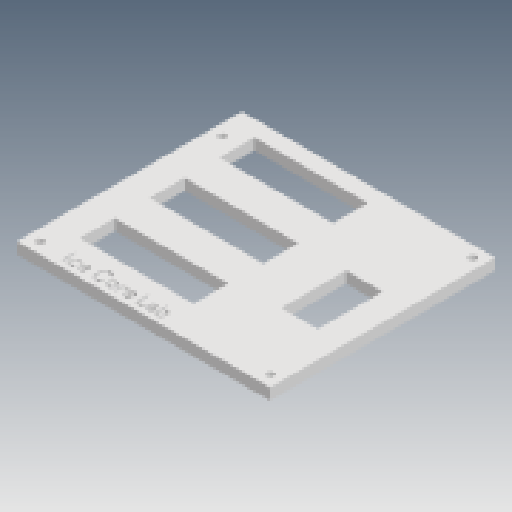
# Autodesk Inventor part: base_plate
Saved by Autodesk Inventor 2025.1 (Build 291241000, 241)
## iProperties
Created: 2026-06-20
Part Number: base_plate
Material: Generic
Document SubType Name: Modeling
Designer: Aiden
Density: 1 g/cm^3
Appearance: Default
Author: Aiden
Autodesk Inventor part; units mm, degrees
ref_plane "YZ Plane" through (0, 0, 0) normal (1, 0, 0) x (0, 1, 0)
ref_plane "XZ Plane" through (0, 0, 0) normal (0, 1, 0) x (-1, 0, 0)
ref_plane "XY Plane" through (0, 0, 0) normal (0, 0, 1) x (1, 0, 0)
sketch "Sketch1" plane through (0, 0, 0) normal (0, 1, 0) x (-1, 0, 0)
  line L0 (112.5, 100) -> (-112.5, 100)
  line L1 (-112.5, 100) -> (-112.5, -100)
  line L2 (-112.5, -100) -> (112.5, -100)
  line L3 (112.5, -100) -> (112.5, 100)
  line L4 (112.5, 100) -> (-112.5, -100) construction
  line L5 (-112.5, 100) -> (112.5, -100) construction
  point P0 (0, 0)
  dimension "d0" = 200
  dimension "d1" = 225
  constraints: 12 end point, 2 midpoint, 2 parallel, 1 horizontal, 1 perpendicular
  measures "d0" distance of L2.end L0.start
  measures "d1" distance of L1.end L2.end
extrude "Extrusion1" add sketch "Sketch1" along normal blind 10
sketch "Sketch3" plane through (0, 10, 0) normal (0, 1, 0) x (1, 0, 0)
  line L0 (-86.9553, 54.5452) -> (13.9553, 54.5452)
  line L1 (13.9553, 54.5452) -> (13.9553, 85.4548)
  line L2 (13.9553, 85.4548) -> (-86.9553, 85.4548)
  line L3 (-86.9553, 85.4548) -> (-86.9553, 54.5452)
  line L4 (-86.9553, 54.5452) -> (13.9553, 85.4548) construction
  line L5 (13.9553, 54.5452) -> (-86.9553, 85.4548) construction
  line L6 (-112.5, 100) -> (-112.5, -100) projected
  line L7 (112.5, 100) -> (-112.5, 100) projected
  line L8 (-86.9553, 23.4548) -> (-86.9553, -7.4548)
  line L9 (-86.9553, -7.4548) -> (13.9553, -7.4548)
  line L10 (13.9553, 23.4548) -> (-86.9553, 23.4548)
  line L11 (13.9553, -7.4548) -> (13.9553, 23.4548)
  line L12 (-86.9553, -38.5452) -> (-86.9553, -69.4548)
  line L13 (-86.9553, -69.4548) -> (13.9553, -69.4548)
  line L14 (13.9553, -38.5452) -> (-86.9553, -38.5452)
  line L15 (13.9553, -69.4548) -> (13.9553, -38.5452)
  point P0 (0, 0)
  point P1 (-36.5, 70)
  dimension "d6" = 76
  dimension "d7" = 30
  dimension "d10" = 62
  constraints: 28 end point, 2 midpoint, 2 parallel, 1 collinear, 1 horizontal, 1 perpendicular, 1 vertical, 15 other
  measures "d6" distance from line of L6 point (-36.5, 70)
  measures "d7" distance from line of L7 point (-36.5, 70)
  measures "d10" distance of L2.end L8.start
extrude "Extrusion3" cut sketch "Sketch3" against normal through all
sketch "Sketch4" plane through (0, 10, 0) normal (0, 1, 0) x (1, 0, 0)
  line L0 (56.2706, -33.7574) -> (88.7294, -33.7574)
  line L1 (88.7294, -33.7574) -> (88.7294, 23.7574)
  line L2 (88.7294, 23.7574) -> (56.2706, 23.7574)
  line L3 (56.2706, 23.7574) -> (56.2706, -33.7574)
  line L4 (56.2706, -33.7574) -> (88.7294, 23.7574) construction
  line L5 (88.7294, -33.7574) -> (56.2706, 23.7574) construction
  line L6 (112.5, -100) -> (112.5, 100) projected
  line L7 (-112.5, -100) -> (112.5, -100) projected
  point P0 (0, 0)
  point P1 (72.5, -5)
  dimension "d17" = 40
  dimension "d18" = 95
  constraints: 12 end point, 2 midpoint, 2 parallel, 1 horizontal, 1 perpendicular
  measures "d17" distance from line of L6 point (72.5, -5)
  measures "d18" distance from line of L7 point (72.5, -5)
extrude "Extrusion4" cut sketch "Sketch4" against normal through all
sketch "Sketch2" plane through (0, 10, 0) normal (0, 1, 0) x (1, 0, 0)
  line L0 (-13.404, -88.2397) -> (-13.404, -81.8012)
  line L1 (-13.404, -81.8012) -> (-13.1143, -82.3338)
  line L2 (-13.1143, -82.3338) -> (-12.6963, -83.0794)
  line L3 (-12.6963, -83.0794) -> (-12.6242, -83.2099)
  line L4 (-12.6242, -83.2099) -> (-12.581, -83.3384)
  line L5 (-12.581, -83.3384) -> (-12.5534, -83.5231)
  line L6 (-12.5534, -83.5231) -> (-12.5284, -83.822)
  line L7 (-12.5284, -83.822) -> (-12.451, -84.7515)
  line L8 (-12.451, -84.7515) -> (-12.3895, -85.418)
  line L9 (-12.3895, -85.418) -> (-12.3583, -85.6558)
  line L10 (-12.3583, -85.6558) -> (-12.3386, -85.6951)
  line L11 (-12.3386, -85.6951) -> (-12.313, -85.6763)
  line L12 (-12.313, -85.6763) -> (-12.2357, -85.4495)
  line L13 (-12.2357, -85.4495) -> (-12.1082, -84.945)
  line L14 (-12.1082, -84.945) -> (-11.9568, -84.3511)
  line L15 (-11.9568, -84.3511) -> (-11.879, -84.1041)
  line L16 (-11.879, -84.1041) -> (-11.6102, -84.3782)
  line L17 (-11.6102, -84.3782) -> (-11.3666, -84.6522)
  line L18 (-11.3666, -84.6522) -> (-11.3476, -88.7862)
  line L19 (-11.3476, -88.7862) -> (-11.3285, -92.9202)
  line L20 (-11.3285, -92.9202) -> (-9.2689, -92.93)
  line L21 (-9.2689, -92.93) -> (-7.2093, -92.9399)
  line L22 (-7.2093, -92.9399) -> (-6.7745, -93.3469)
  line L23 (-6.7745, -93.3469) -> (-5.8675, -94.2035)
  line L24 (-5.8675, -94.2035) -> (-5.3953, -94.6529)
  line L25 (-5.3953, -94.6529) -> (-9.314, -94.6561)
  line L26 (-9.314, -94.6561) -> (-13.3183, -94.6688)
  line L27 (-13.3183, -94.6688) -> (-13.3466, -94.6593)
  line L28 (-13.3466, -94.6593) -> (-13.3679, -94.5737)
  line L29 (-13.3679, -94.5737) -> (-13.3933, -93.8723)
  line L30 (-13.3933, -93.8723) -> (-13.404, -88.2397)
  line L31 (-3.7121, -94.6461) -> (-4.5026, -93.8769)
  line L32 (-4.5026, -93.8769) -> (-5.255, -93.1487)
  line L33 (-5.255, -93.1487) -> (-5.2617, -92.2745)
  line L34 (-5.2617, -92.2745) -> (-5.2684, -91.4003)
  line L35 (-5.2684, -91.4003) -> (-4.4522, -90.6105)
  line L36 (-4.4522, -90.6105) -> (-3.7551, -89.9567)
  line L37 (-3.7551, -89.9567) -> (-3.5944, -89.8366)
  line L38 (-3.5944, -89.8366) -> (-3.4895, -89.7956)
  line L39 (-3.4895, -89.7956) -> (-2.9007, -89.7861)
  line L40 (-2.9007, -89.7861) -> (-1.6907, -89.7986)
  line L41 (-1.6907, -89.7986) -> (-0.4099, -89.8104)
  line L42 (-0.4099, -89.8104) -> (-0.103, -89.8024)
  line L43 (-0.103, -89.8024) -> (0.0122, -89.7849)
  line L44 (0.0122, -89.7849) -> (0.0351, -89.7449)
  line L45 (0.0351, -89.7449) -> (0.0486, -89.6654)
  line L46 (0.0486, -89.6654) -> (0.0502, -89.3514)
  line L47 (0.0502, -89.3514) -> (0.0379, -88.9596)
  line L48 (0.0379, -88.9596) -> (-0.2049, -88.7216)
  line L49 (-0.2049, -88.7216) -> (-0.3755, -88.56)
  line L50 (-0.3755, -88.56) -> (-0.4725, -88.4999)
  line L51 (-0.4725, -88.4999) -> (-0.5035, -88.5064)
  line L52 (-0.5035, -88.5064) -> (-0.5284, -88.5365)
  line L53 (-0.5284, -88.5365) -> (-0.5762, -88.6645)
  line L54 (-0.5762, -88.6645) -> (-0.6336, -88.8454)
  line L55 (-0.6336, -88.8454) -> (-0.6972, -88.5713)
  line L56 (-0.6972, -88.5713) -> (-0.7446, -88.3459)
  line L57 (-0.7446, -88.3459) -> (-0.7467, -88.2043)
  line L58 (-0.7467, -88.2043) -> (-0.6919, -88.0906)
  line L59 (-0.6919, -88.0906) -> (-0.5686, -87.9487)
  line L60 (-0.5686, -87.9487) -> (-0.4266, -87.7773)
  line L61 (-0.4266, -87.7773) -> (-0.309, -87.5863)
  line L62 (-0.309, -87.5863) -> (-0.1974, -87.3407)
  line L63 (-0.1974, -87.3407) -> (-0.0732, -87.0052)
  line L64 (-0.0732, -87.0052) -> (0.0505, -86.6503)
  line L65 (0.0505, -86.6503) -> (0.2762, -86.8719)
  line L66 (0.2762, -86.8719) -> (0.5441, -87.1421)
  line L67 (0.5441, -87.1421) -> (0.6264, -87.2474)
  line L68 (0.6264, -87.2474) -> (0.6836, -87.3559)
  line L69 (0.6836, -87.3559) -> (0.7228, -87.485)
  line L70 (0.7228, -87.485) -> (0.751, -87.6519)
  line L71 (0.751, -87.6519) -> (0.8024, -88.1684)
  line L72 (0.8024, -88.1684) -> (0.8995, -89.1458)
  line L73 (0.8995, -89.1458) -> (0.9268, -89.3166)
  line L74 (0.9268, -89.3166) -> (0.9503, -89.3595)
  line L75 (0.9503, -89.3595) -> (1.0112, -89.1612)
  line L76 (1.0112, -89.1612) -> (1.1203, -88.6845)
  line L77 (1.1203, -88.6845) -> (1.2844, -87.976)
  line L78 (1.2844, -87.976) -> (1.3146, -87.9851)
  line L79 (1.3146, -87.9851) -> (1.3816, -88.0344)
  line L80 (1.3816, -88.0344) -> (1.586, -88.2217)
  line L81 (1.586, -88.2217) -> (1.867, -88.5007)
  line L82 (1.867, -88.5007) -> (1.867, -91.5959)
  line L83 (1.867, -91.5959) -> (1.867, -94.691)
  line L84 (1.867, -94.691) -> (-0.9035, -94.6891)
  line L85 (-0.9035, -94.6891) -> (-3.0215, -94.6779)
  line L86 (-3.0215, -94.6779) -> (-3.5334, -94.6647)
  line L87 (-3.5334, -94.6647) -> (-3.7121, -94.6461)
  line L88 (-3.7121, -94.6461) -> (-3.7121, -94.6461)
  line L89 (0.039, -92.2728) -> (0.039, -91.4159)
  line L90 (0.039, -91.4159) -> (-1.5308, -91.4159)
  line L91 (-1.5308, -91.4159) -> (-3.1007, -91.4159)
  line L92 (-3.1007, -91.4159) -> (-3.3397, -91.6528)
  line L93 (-3.3397, -91.6528) -> (-3.5788, -91.8898)
  line L94 (-3.5788, -91.8898) -> (-3.5788, -92.2779)
  line L95 (-3.5788, -92.2779) -> (-3.5788, -92.666)
  line L96 (-3.5788, -92.666) -> (-3.3217, -92.8971)
  line L97 (-3.3217, -92.8971) -> (-3.0647, -93.1282)
  line L98 (-3.0647, -93.1282) -> (-1.5128, -93.1289)
  line L99 (-1.5128, -93.1289) -> (0.039, -93.1296)
  line L100 (0.039, -93.1296) -> (0.039, -92.2728)
  line L101 (3.5045, -88.2678) -> (3.5091, -83.7361)
  line L102 (3.5091, -83.7361) -> (3.52, -81.8604)
  line L103 (3.52, -81.8604) -> (3.849, -82.4264)
  line L104 (3.849, -82.4264) -> (4.2849, -83.169)
  line L105 (4.2849, -83.169) -> (4.3551, -83.2892)
  line L106 (4.3551, -83.2892) -> (4.3945, -83.412)
  line L107 (4.3945, -83.412) -> (4.416, -83.6042)
  line L108 (4.416, -83.6042) -> (4.4326, -83.9328)
  line L109 (4.4326, -83.9328) -> (4.5137, -85.2495)
  line L110 (4.5137, -85.2495) -> (4.5555, -85.6202)
  line L111 (4.5555, -85.6202) -> (4.5748, -85.7119)
  line L112 (4.5748, -85.7119) -> (4.5923, -85.7329)
  line L113 (4.5923, -85.7329) -> (4.7768, -85.0905)
  line L114 (4.7768, -85.0905) -> (4.9883, -84.2999)
  line L115 (4.9883, -84.2999) -> (5.033, -84.1339)
  line L116 (5.033, -84.1339) -> (5.2303, -84.3908)
  line L117 (5.2303, -84.3908) -> (5.4277, -84.6476)
  line L118 (5.4277, -84.6476) -> (5.4484, -85.7373)
  line L119 (5.4484, -85.7373) -> (5.4692, -86.827)
  line L120 (5.4692, -86.827) -> (5.696, -87.5286)
  line L121 (5.696, -87.5286) -> (5.8706, -88.0288)
  line L122 (5.8706, -88.0288) -> (5.972, -88.2463)
  line L123 (5.972, -88.2463) -> (6.0026, -88.251)
  line L124 (6.0026, -88.251) -> (6.0024, -88.1902)
  line L125 (6.0024, -88.1902) -> (5.8625, -87.5887)
  line L126 (5.8625, -87.5887) -> (5.768, -87.1659)
  line L127 (5.768, -87.1659) -> (5.7229, -86.8803)
  line L128 (5.7229, -86.8803) -> (5.7258, -86.7162)
  line L129 (5.7258, -86.7162) -> (5.7448, -86.6749)
  line L130 (5.7448, -86.6749) -> (5.7752, -86.6581)
  line L131 (5.7752, -86.6581) -> (6.3687, -86.6426)
  line L132 (6.3687, -86.6426) -> (7.4599, -86.642)
  line L133 (7.4599, -86.642) -> (8.5168, -86.6536)
  line L134 (8.5168, -86.6536) -> (9.0072, -86.6747)
  line L135 (9.0072, -86.6747) -> (9.9345, -87.6153)
  line L136 (9.9345, -87.6153) -> (10.8163, -88.5178)
  line L137 (10.8163, -88.5178) -> (10.8163, -90.7417)
  line L138 (10.8163, -90.7417) -> (10.8163, -92.9656)
  line L139 (10.8163, -92.9656) -> (9.9422, -93.8283)
  line L140 (9.9422, -93.8283) -> (9.068, -94.691)
  line L141 (9.068, -94.691) -> (6.2863, -94.691)
  line L142 (6.2863, -94.691) -> (3.5045, -94.691)
  line L143 (3.5045, -94.691) -> (3.5045, -88.2678)
  line L144 (8.7875, -92.8155) -> (9.0607, -92.5394)
  line L145 (9.0607, -92.5394) -> (9.068, -90.6986)
  line L146 (9.068, -90.6986) -> (9.0753, -88.8579)
  line L147 (9.0753, -88.8579) -> (8.7757, -88.5565)
  line L148 (8.7757, -88.5565) -> (8.4761, -88.2551)
  line L149 (8.4761, -88.2551) -> (7.3993, -88.2551)
  line L150 (7.3993, -88.2551) -> (6.3226, -88.2551)
  line L151 (6.3226, -88.2551) -> (6.3226, -87.6966)
  line L152 (6.3226, -87.6966) -> (6.3179, -87.3068)
  line L153 (6.3179, -87.3068) -> (6.3066, -87.1541)
  line L154 (6.3066, -87.1541) -> (6.1898, -87.7983)
  line L155 (6.1898, -87.7983) -> (6.0571, -88.582)
  line L156 (6.0571, -88.582) -> (6.0315, -88.6697)
  line L157 (6.0315, -88.6697) -> (6.022, -88.6074)
  line L158 (6.022, -88.6074) -> (6.0098, -88.5153)
  line L159 (6.0098, -88.5153) -> (5.9931, -88.4973)
  line L160 (5.9931, -88.4973) -> (5.9652, -88.4997)
  line L161 (5.9652, -88.4997) -> (5.8634, -88.5697)
  line L162 (5.8634, -88.5697) -> (5.6799, -88.7347)
  line L163 (5.6799, -88.7347) -> (5.4086, -88.9858)
  line L164 (5.4086, -88.9858) -> (5.4086, -91.0387)
  line L165 (5.4086, -91.0387) -> (5.4086, -93.0916)
  line L166 (5.4086, -93.0916) -> (6.9615, -93.0916)
  line L167 (6.9615, -93.0916) -> (8.5143, -93.0916)
  line L168 (8.5143, -93.0916) -> (8.7875, -92.8155)
  line L169 (-78.5874, -88.2555) -> (-78.575, -83.2395)
  line L170 (-78.575, -83.2395) -> (-78.5608, -82.1971)
  line L171 (-78.5608, -82.1971) -> (-78.551, -81.968)
  line L172 (-78.551, -81.968) -> (-78.5394, -81.9053)
  line L173 (-78.5394, -81.9053) -> (-78.1054, -82.5808)
  line L174 (-78.1054, -82.5808) -> (-77.6681, -83.2663)
  line L175 (-77.6681, -83.2663) -> (-77.6355, -83.3847)
  line L176 (-77.6355, -83.3847) -> (-77.6081, -83.7115)
  line L177 (-77.6081, -83.7115) -> (-77.548, -85.3513)
  line L178 (-77.548, -85.3513) -> (-77.5219, -85.9498)
  line L179 (-77.5219, -85.9498) -> (-77.4947, -86.1987)
  line L180 (-77.4947, -86.1987) -> (-77.462, -86.1436)
  line L181 (-77.462, -86.1436) -> (-77.4003, -85.9434)
  line L182 (-77.4003, -85.9434) -> (-77.1315, -84.8971)
  line L183 (-77.1315, -84.8971) -> (-77.0176, -84.4488)
  line L184 (-77.0176, -84.4488) -> (-76.9774, -84.3266)
  line L185 (-76.9774, -84.3266) -> (-76.9401, -84.2654)
  line L186 (-76.9401, -84.2654) -> (-76.8995, -84.2597)
  line L187 (-76.8995, -84.2597) -> (-76.8495, -84.3043)
  line L188 (-76.8495, -84.3043) -> (-76.6964, -84.523)
  line L189 (-76.6964, -84.523) -> (-76.5559, -84.6868)
  line L190 (-76.5559, -84.6868) -> (-76.5312, -84.9107)
  line L191 (-76.5312, -84.9107) -> (-76.5161, -85.6819)
  line L192 (-76.5161, -85.6819) -> (-76.5064, -89.6851)
  line L193 (-76.5064, -89.6851) -> (-76.5064, -94.6529)
  line L194 (-76.5064, -94.6529) -> (-77.5487, -94.6529)
  line L195 (-77.5487, -94.6529) -> (-78.591, -94.6529)
  line L196 (-78.591, -94.6529) -> (-78.5874, -88.2555)
  line L197 (-73.7822, -93.6433) -> (-74.7927, -92.6337)
  line L198 (-74.7927, -92.6337) -> (-74.7927, -90.5489)
  line L199 (-74.7927, -90.5489) -> (-74.7927, -88.464)
  line L200 (-74.7927, -88.464) -> (-73.804, -87.4759)
  line L201 (-73.804, -87.4759) -> (-73.1012, -86.7831)
  line L202 (-73.1012, -86.7831) -> (-72.8, -86.505)
  line L203 (-72.8, -86.505) -> (-72.7258, -86.7061)
  line L204 (-72.7258, -86.7061) -> (-72.6022, -87.1442)
  line L205 (-72.6022, -87.1442) -> (-72.3282, -88.2761)
  line L206 (-72.3282, -88.2761) -> (-72.3364, -88.328)
  line L207 (-72.3364, -88.328) -> (-72.3873, -88.4004)
  line L208 (-72.3873, -88.4004) -> (-72.6571, -88.6524)
  line L209 (-72.6571, -88.6524) -> (-73.0028, -88.9505)
  line L210 (-73.0028, -88.9505) -> (-73.0028, -90.5361)
  line L211 (-73.0028, -90.5361) -> (-73.0028, -92.1217)
  line L212 (-73.0028, -92.1217) -> (-72.5734, -92.5499)
  line L213 (-72.5734, -92.5499) -> (-72.1439, -92.9782)
  line L214 (-72.1439, -92.9782) -> (-70.5836, -92.9682)
  line L215 (-70.5836, -92.9682) -> (-69.0232, -92.9583)
  line L216 (-69.0232, -92.9583) -> (-69.0042, -92.6346)
  line L217 (-69.0042, -92.6346) -> (-68.9852, -92.3109)
  line L218 (-68.9852, -92.3109) -> (-68.5349, -92.7471)
  line L219 (-68.5349, -92.7471) -> (-67.3787, -93.9181)
  line L220 (-67.3787, -93.9181) -> (-66.6727, -94.6529)
  line L221 (-66.6727, -94.6529) -> (-69.7221, -94.6529)
  line L222 (-69.7221, -94.6529) -> (-72.7716, -94.6529)
  line L223 (-72.7716, -94.6529) -> (-73.7822, -93.6433)
  line L224 (-64.7678, -93.7291) -> (-65.691, -92.8054)
  line L225 (-65.691, -92.8054) -> (-65.691, -90.5591)
  line L226 (-65.691, -90.5591) -> (-65.691, -88.3129)
  line L227 (-65.691, -88.3129) -> (-64.9046, -87.5258)
  line L228 (-64.9046, -87.5258) -> (-64.3363, -86.9748)
  line L229 (-64.3363, -86.9748) -> (-64.1533, -86.811)
  line L230 (-64.1533, -86.811) -> (-64.0743, -86.7555)
  line L231 (-64.0743, -86.7555) -> (-63.9764, -86.7563)
  line L232 (-63.9764, -86.7563) -> (-63.8698, -86.7077)
  line L233 (-63.8698, -86.7077) -> (-63.784, -86.6294)
  line L234 (-63.784, -86.6294) -> (-63.7488, -86.5409)
  line L235 (-63.7488, -86.5409) -> (-63.7488, -86.4272)
  line L236 (-63.7488, -86.4272) -> (-62.0161, -86.4272)
  line L237 (-62.0161, -86.4272) -> (-60.4999, -86.4379)
  line L238 (-60.4999, -86.4379) -> (-60.3102, -86.4633)
  line L239 (-60.3102, -86.4633) -> (-60.2863, -86.4846)
  line L240 (-60.2863, -86.4846) -> (-60.2828, -86.5128)
  line L241 (-60.2828, -86.5128) -> (-60.2714, -86.605)
  line L242 (-60.2714, -86.605) -> (-60.2367, -86.6623)
  line L243 (-60.2367, -86.6623) -> (-60.1752, -86.6875)
  line L244 (-60.1752, -86.6875) -> (-60.0835, -86.6836)
  line L245 (-60.0835, -86.6836) -> (-59.9938, -86.6866)
  line L246 (-59.9938, -86.6866) -> (-59.8624, -86.7726)
  line L247 (-59.8624, -86.7726) -> (-59.6074, -87.0104)
  line L248 (-59.6074, -87.0104) -> (-59.1467, -87.4686)
  line L249 (-59.1467, -87.4686) -> (-58.3411, -88.2748)
  line L250 (-58.3411, -88.2748) -> (-58.3411, -89.7882)
  line L251 (-58.3411, -89.7882) -> (-58.3411, -91.3017)
  line L252 (-58.3411, -91.3017) -> (-61.1192, -91.3017)
  line L253 (-61.1192, -91.3017) -> (-63.8972, -91.3017)
  line L254 (-63.8972, -91.3017) -> (-63.9087, -91.8634)
  line L255 (-63.9087, -91.8634) -> (-63.907, -92.2397)
  line L256 (-63.907, -92.2397) -> (-63.8909, -92.3696)
  line L257 (-63.8909, -92.3696) -> (-63.8589, -92.4744)
  line L258 (-63.8589, -92.4744) -> (-63.8064, -92.564)
  line L259 (-63.8064, -92.564) -> (-63.7291, -92.6488)
  line L260 (-63.7291, -92.6488) -> (-63.4822, -92.844)
  line L261 (-63.4822, -92.844) -> (-63.3007, -92.9773)
  line L262 (-63.3007, -92.9773) -> (-60.8308, -92.9773)
  line L263 (-60.8308, -92.9773) -> (-58.3608, -92.9773)
  line L264 (-58.3608, -92.9773) -> (-59.198, -93.8151)
  line L265 (-59.198, -93.8151) -> (-60.0352, -94.6529)
  line L266 (-60.0352, -94.6529) -> (-61.9399, -94.6529)
  line L267 (-61.9399, -94.6529) -> (-63.8446, -94.6529)
  line L268 (-63.8446, -94.6529) -> (-64.7678, -93.7291)
  line L269 (-60.1396, -89.018) -> (-60.1347, -88.5362)
  line L270 (-60.1347, -88.5362) -> (-60.1497, -88.3018)
  line L271 (-60.1497, -88.3018) -> (-60.1701, -88.2538)
  line L272 (-60.1701, -88.2538) -> (-60.2019, -88.2395)
  line L273 (-60.2019, -88.2395) -> (-60.3083, -88.2742)
  line L274 (-60.3083, -88.2742) -> (-60.3911, -88.3059)
  line L275 (-60.3911, -88.3059) -> (-60.4464, -88.3105)
  line L276 (-60.4464, -88.3105) -> (-60.4975, -88.2829)
  line L277 (-60.4975, -88.2829) -> (-60.568, -88.2179)
  line L278 (-60.568, -88.2179) -> (-60.6569, -88.1513)
  line L279 (-60.6569, -88.1513) -> (-60.8338, -88.1172)
  line L280 (-60.8338, -88.1172) -> (-61.2311, -88.1046)
  line L281 (-61.2311, -88.1046) -> (-61.9813, -88.1028)
  line L282 (-61.9813, -88.1028) -> (-63.2757, -88.1028)
  line L283 (-63.2757, -88.1028) -> (-63.4612, -88.2912)
  line L284 (-63.4612, -88.2912) -> (-63.57, -88.3989)
  line L285 (-63.57, -88.3989) -> (-63.6354, -88.4467)
  line L286 (-63.6354, -88.4467) -> (-63.6836, -88.4453)
  line L287 (-63.6836, -88.4453) -> (-63.741, -88.4054)
  line L288 (-63.741, -88.4054) -> (-63.8529, -88.3323)
  line L289 (-63.8529, -88.3323) -> (-63.8873, -88.3352)
  line L290 (-63.8873, -88.3352) -> (-63.9097, -88.3726)
  line L291 (-63.9097, -88.3726) -> (-63.926, -88.575)
  line L292 (-63.926, -88.575) -> (-63.9164, -88.9882)
  line L293 (-63.9164, -88.9882) -> (-63.88, -89.6931)
  line L294 (-63.88, -89.6931) -> (-63.7888, -89.7161)
  line L295 (-63.7888, -89.7161) -> (-63.4896, -89.7292)
  line L296 (-63.4896, -89.7292) -> (-62.0076, -89.7312)
  line L297 (-62.0076, -89.7312) -> (-60.1501, -89.7213)
  line L298 (-60.1501, -89.7213) -> (-60.1396, -89.018)
  line L299 (-51.5382, -93.2441) -> (-52.9335, -91.8352)
  line L300 (-52.9335, -91.8352) -> (-52.9335, -88.3045)
  line L301 (-52.9335, -88.3045) -> (-52.9335, -84.7737)
  line L302 (-52.9335, -84.7737) -> (-52.3908, -84.2198)
  line L303 (-52.3908, -84.2198) -> (-51.235, -83.0182)
  line L304 (-51.235, -83.0182) -> (-50.8409, -82.6214)
  line L305 (-50.8409, -82.6214) -> (-50.5018, -82.3165)
  line L306 (-50.5018, -82.3165) -> (-50.2526, -82.1325)
  line L307 (-50.2526, -82.1325) -> (-50.1726, -82.0949)
  line L308 (-50.1726, -82.0949) -> (-50.1282, -82.0983)
  line L309 (-50.1282, -82.0983) -> (-50.0064, -82.4889)
  line L310 (-50.0064, -82.4889) -> (-49.8709, -82.9426)
  line L311 (-49.8709, -82.9426) -> (-49.8662, -82.962)
  line L312 (-49.8662, -82.962) -> (-49.8734, -82.9584)
  line L313 (-49.8734, -82.9584) -> (-49.9169, -82.8895)
  line L314 (-49.9169, -82.8895) -> (-49.9745, -82.8082)
  line L315 (-49.9745, -82.8082) -> (-49.9968, -82.7912)
  line L316 (-49.9968, -82.7912) -> (-50.0106, -82.7943)
  line L317 (-50.0106, -82.7943) -> (-50.0615, -82.9696)
  line L318 (-50.0615, -82.9696) -> (-50.1409, -83.3275)
  line L319 (-50.1409, -83.3275) -> (-50.2936, -84.1519)
  line L320 (-50.2936, -84.1519) -> (-50.3367, -84.4138)
  line L321 (-50.3367, -84.4138) -> (-50.383, -84.5683)
  line L322 (-50.383, -84.5683) -> (-50.4613, -84.6759)
  line L323 (-50.4613, -84.6759) -> (-50.6003, -84.797)
  line L324 (-50.6003, -84.797) -> (-50.8389, -84.9944)
  line L325 (-50.8389, -84.9944) -> (-50.8389, -88.2589)
  line L326 (-50.8389, -88.2589) -> (-50.8389, -91.5235)
  line L327 (-50.8389, -91.5235) -> (-50.1847, -92.1552)
  line L328 (-50.1847, -92.1552) -> (-49.5305, -92.7869)
  line L329 (-49.5305, -92.7869) -> (-47.7604, -92.7869)
  line L330 (-47.7604, -92.7869) -> (-45.9902, -92.7869)
  line L331 (-45.9902, -92.7869) -> (-45.4346, -92.2457)
  line L332 (-45.4346, -92.2457) -> (-44.879, -91.7045)
  line L333 (-44.879, -91.7045) -> (-43.737, -91.7153)
  line L334 (-43.737, -91.7153) -> (-42.5856, -91.7354)
  line L335 (-42.5856, -91.7354) -> (-42.7007, -91.8835)
  line L336 (-42.7007, -91.8835) -> (-43.0528, -92.263)
  line L337 (-43.0528, -92.263) -> (-44.2995, -93.539)
  line L338 (-44.2995, -93.539) -> (-45.4077, -94.6529)
  line L339 (-45.4077, -94.6529) -> (-47.7753, -94.6529)
  line L340 (-47.7753, -94.6529) -> (-50.1429, -94.6529)
  line L341 (-50.1429, -94.6529) -> (-51.5382, -93.2441)
  line L342 (-40.2809, -93.653) -> (-41.2803, -92.6531)
  line L343 (-41.2803, -92.6531) -> (-41.2786, -90.5207)
  line L344 (-41.2786, -90.5207) -> (-41.2768, -88.3884)
  line L345 (-41.2768, -88.3884) -> (-40.4669, -87.5585)
  line L346 (-40.4669, -87.5585) -> (-39.8183, -86.9137)
  line L347 (-39.8183, -86.9137) -> (-39.6635, -86.7832)
  line L348 (-39.6635, -86.7832) -> (-39.5923, -86.7536)
  line L349 (-39.5923, -86.7536) -> (-39.5294, -86.7569)
  line L350 (-39.5294, -86.7569) -> (-39.4693, -86.7301)
  line L351 (-39.4693, -86.7301) -> (-39.4187, -86.7049)
  line L352 (-39.4187, -86.7049) -> (-39.3802, -86.7163)
  line L353 (-39.3802, -86.7163) -> (-39.2931, -86.9778)
  line L354 (-39.2931, -86.9778) -> (-39.1498, -87.5091)
  line L355 (-39.1498, -87.5091) -> (-39.016, -88.0541)
  line L356 (-39.016, -88.0541) -> (-38.9577, -88.3571)
  line L357 (-38.9577, -88.3571) -> (-39.0306, -88.4394)
  line L358 (-39.0306, -88.4394) -> (-39.2052, -88.5933)
  line L359 (-39.2052, -88.5933) -> (-39.4523, -88.7982)
  line L360 (-39.4523, -88.7982) -> (-39.4523, -90.4821)
  line L361 (-39.4523, -90.4821) -> (-39.4523, -92.1659)
  line L362 (-39.4523, -92.1659) -> (-39.0681, -92.5525)
  line L363 (-39.0681, -92.5525) -> (-38.6838, -92.9392)
  line L364 (-38.6838, -92.9392) -> (-37.3258, -92.9392)
  line L365 (-37.3258, -92.9392) -> (-35.9678, -92.9392)
  line L366 (-35.9678, -92.9392) -> (-35.5979, -92.5489)
  line L367 (-35.5979, -92.5489) -> (-35.2281, -92.1585)
  line L368 (-35.2281, -92.1585) -> (-35.2262, -90.4448)
  line L369 (-35.2262, -90.4448) -> (-35.2244, -88.7311)
  line L370 (-35.2244, -88.7311) -> (-35.5724, -88.3979)
  line L371 (-35.5724, -88.3979) -> (-35.9204, -88.0647)
  line L372 (-35.9204, -88.0647) -> (-37.1886, -88.0647)
  line L373 (-37.1886, -88.0647) -> (-38.0049, -88.067)
  line L374 (-38.0049, -88.067) -> (-38.249, -88.0762)
  line L375 (-38.249, -88.0762) -> (-38.4099, -88.0966)
  line L376 (-38.4099, -88.0966) -> (-38.5074, -88.1324)
  line L377 (-38.5074, -88.1324) -> (-38.5611, -88.188)
  line L378 (-38.5611, -88.188) -> (-38.5907, -88.2674)
  line L379 (-38.5907, -88.2674) -> (-38.6159, -88.3752)
  line L380 (-38.6159, -88.3752) -> (-38.6637, -88.5743)
  line L381 (-38.6637, -88.5743) -> (-38.7515, -88.1386)
  line L382 (-38.7515, -88.1386) -> (-38.8756, -87.6418)
  line L383 (-38.8756, -87.6418) -> (-39.0506, -87.0593)
  line L384 (-39.0506, -87.0593) -> (-39.2619, -86.4024)
  line L385 (-39.2619, -86.4024) -> (-37.3102, -86.3887)
  line L386 (-37.3102, -86.3887) -> (-35.3585, -86.3883)
  line L387 (-35.3585, -86.3883) -> (-34.3972, -87.3693)
  line L388 (-34.3972, -87.3693) -> (-33.4359, -88.3503)
  line L389 (-33.4359, -88.3503) -> (-33.4356, -90.511)
  line L390 (-33.4356, -90.511) -> (-33.4353, -92.6717)
  line L391 (-33.4353, -92.6717) -> (-34.3969, -93.6578)
  line L392 (-34.3969, -93.6578) -> (-35.3585, -94.6439)
  line L393 (-35.3585, -94.6439) -> (-37.32, -94.6484)
  line L394 (-37.32, -94.6484) -> (-39.2815, -94.6529)
  line L395 (-39.2815, -94.6529) -> (-40.2809, -93.653)
  line L396 (-31.7123, -90.5305) -> (-31.7026, -86.4081)
  line L397 (-31.7026, -86.4081) -> (-31.3449, -86.4081)
  line L398 (-31.3449, -86.4081) -> (-31.1773, -86.4071)
  line L399 (-31.1773, -86.4071) -> (-31.053, -86.4169)
  line L400 (-31.053, -86.4169) -> (-30.9635, -86.4562)
  line L401 (-30.9635, -86.4562) -> (-30.9005, -86.5441)
  line L402 (-30.9005, -86.5441) -> (-30.8555, -86.6994)
  line L403 (-30.8555, -86.6994) -> (-30.8203, -86.9412)
  line L404 (-30.8203, -86.9412) -> (-30.7451, -87.7598)
  line L405 (-30.7451, -87.7598) -> (-30.6951, -88.1268)
  line L406 (-30.6951, -88.1268) -> (-30.6689, -88.1966)
  line L407 (-30.6689, -88.1966) -> (-30.6564, -88.1993)
  line L408 (-30.6564, -88.1993) -> (-30.6447, -88.1789)
  line L409 (-30.6447, -88.1789) -> (-30.4814, -87.5419)
  line L410 (-30.4814, -87.5419) -> (-30.338, -86.9619)
  line L411 (-30.338, -86.9619) -> (-30.2206, -87.032)
  line L412 (-30.2206, -87.032) -> (-29.9088, -87.2071)
  line L413 (-29.9088, -87.2071) -> (-29.8517, -87.2209)
  line L414 (-29.8517, -87.2209) -> (-29.8248, -87.2007)
  line L415 (-29.8248, -87.2007) -> (-29.4932, -86.7938)
  line L416 (-29.4932, -86.7938) -> (-29.1891, -86.4314)
  line L417 (-29.1891, -86.4314) -> (-28.8845, -86.4218)
  line L418 (-28.8845, -86.4218) -> (-26.8665, -86.4105)
  line L419 (-26.8665, -86.4105) -> (-25.2477, -86.4246)
  line L420 (-25.2477, -86.4246) -> (-26.0569, -87.2529)
  line L421 (-26.0569, -87.2529) -> (-26.8661, -88.0646)
  line L422 (-26.8661, -88.0646) -> (-27.933, -88.0646)
  line L423 (-27.933, -88.0646) -> (-29, -88.0647)
  line L424 (-29, -88.0647) -> (-29.4278, -88.4937)
  line L425 (-29.4278, -88.4937) -> (-29.8556, -88.9227)
  line L426 (-29.8556, -88.9227) -> (-29.8556, -91.7878)
  line L427 (-29.8556, -91.7878) -> (-29.8556, -94.6529)
  line L428 (-29.8556, -94.6529) -> (-30.7888, -94.6529)
  line L429 (-30.7888, -94.6529) -> (-31.7219, -94.6529)
  line L430 (-31.7219, -94.6529) -> (-31.7123, -90.5305)
  line L431 (-24.3828, -93.7281) -> (-25.3269, -92.8059)
  line L432 (-25.3269, -92.8059) -> (-25.3251, -90.5781)
  line L433 (-25.3251, -90.5781) -> (-25.3233, -88.3503)
  line L434 (-25.3233, -88.3503) -> (-24.555, -87.5752)
  line L435 (-24.555, -87.5752) -> (-24.13, -87.1502)
  line L436 (-24.13, -87.1502) -> (-23.8722, -86.9088)
  line L437 (-23.8722, -86.9088) -> (-23.7107, -86.7901)
  line L438 (-23.7107, -86.7901) -> (-23.5747, -86.7331)
  line L439 (-23.5747, -86.7331) -> (-23.4598, -86.6936)
  line L440 (-23.4598, -86.6936) -> (-23.3944, -86.6578)
  line L441 (-23.3944, -86.6578) -> (-23.3631, -86.6131)
  line L442 (-23.3631, -86.6131) -> (-23.3506, -86.5467)
  line L443 (-23.3506, -86.5467) -> (-23.3387, -86.4272)
  line L444 (-23.3387, -86.4272) -> (-21.5957, -86.4272)
  line L445 (-21.5957, -86.4272) -> (-19.8528, -86.4272)
  line L446 (-19.8528, -86.4272) -> (-19.6892, -86.57)
  line L447 (-19.6892, -86.57) -> (-18.7307, -87.4923)
  line L448 (-18.7307, -87.4923) -> (-17.9358, -88.2717)
  line L449 (-17.9358, -88.2717) -> (-17.9358, -89.7865)
  line L450 (-17.9358, -89.7865) -> (-17.9358, -91.3012)
  line L451 (-17.9358, -91.3012) -> (-20.7253, -91.311)
  line L452 (-20.7253, -91.311) -> (-23.5149, -91.3207)
  line L453 (-23.5149, -91.3207) -> (-23.5254, -91.8781)
  line L454 (-23.5254, -91.8781) -> (-23.5359, -92.4355)
  line L455 (-23.5359, -92.4355) -> (-23.2439, -92.6969)
  line L456 (-23.2439, -92.6969) -> (-22.9519, -92.9583)
  line L457 (-22.9519, -92.9583) -> (-20.4613, -92.9773)
  line L458 (-20.4613, -92.9773) -> (-17.9708, -92.9963)
  line L459 (-17.9708, -92.9963) -> (-18.8007, -93.8245)
  line L460 (-18.8007, -93.8245) -> (-19.6305, -94.6527)
  line L461 (-19.6305, -94.6527) -> (-21.5346, -94.6515)
  line L462 (-21.5346, -94.6515) -> (-23.4387, -94.6504)
  line L463 (-23.4387, -94.6504) -> (-24.3828, -93.7281)
  line L464 (-19.7487, -89.7086) -> (-19.7307, -89.4632)
  line L465 (-19.7307, -89.4632) -> (-19.7203, -88.9651)
  line L466 (-19.7203, -88.9651) -> (-19.7201, -88.4704)
  line L467 (-19.7201, -88.4704) -> (-19.7331, -88.235)
  line L468 (-19.7331, -88.235) -> (-19.7913, -88.2369)
  line L469 (-19.7913, -88.2369) -> (-19.8997, -88.2728)
  line L470 (-19.8997, -88.2728) -> (-19.9847, -88.3056)
  line L471 (-19.9847, -88.3056) -> (-20.0407, -88.3107)
  line L472 (-20.0407, -88.3107) -> (-20.092, -88.2832)
  line L473 (-20.092, -88.2832) -> (-20.1627, -88.2179)
  line L474 (-20.1627, -88.2179) -> (-20.2517, -88.1513)
  line L475 (-20.2517, -88.1513) -> (-20.4291, -88.1172)
  line L476 (-20.4291, -88.1172) -> (-20.8278, -88.1046)
  line L477 (-20.8278, -88.1046) -> (-21.5809, -88.1028)
  line L478 (-21.5809, -88.1028) -> (-22.8804, -88.1028)
  line L479 (-22.8804, -88.1028) -> (-23.0906, -88.2949)
  line L480 (-23.0906, -88.2949) -> (-23.2791, -88.4477)
  line L481 (-23.2791, -88.4477) -> (-23.3306, -88.4587)
  line L482 (-23.3306, -88.4587) -> (-23.3784, -88.4387)
  line L483 (-23.3784, -88.4387) -> (-23.4289, -88.4127)
  line L484 (-23.4289, -88.4127) -> (-23.4685, -88.4083)
  line L485 (-23.4685, -88.4083) -> (-23.4984, -88.4298)
  line L486 (-23.4984, -88.4298) -> (-23.5194, -88.4817)
  line L487 (-23.5194, -88.4817) -> (-23.5399, -88.6946)
  line L488 (-23.5399, -88.6946) -> (-23.5389, -89.0826)
  line L489 (-23.5389, -89.0826) -> (-23.5097, -89.7106)
  line L490 (-23.5097, -89.7106) -> (-22.9151, -89.7329)
  line L491 (-22.9151, -89.7329) -> (-21.6292, -89.7397)
  line L492 (-21.6292, -89.7397) -> (-20.3433, -89.7315)
  line L493 (-20.3433, -89.7315) -> (-19.7487, -89.7086)
  line L494 (-72.0634, -88.7883) -> (-72.2, -88.1409)
  line L495 (-72.2, -88.1409) -> (-72.3253, -87.559)
  line L496 (-72.3253, -87.559) -> (-72.4652, -86.9889)
  line L497 (-72.4652, -86.9889) -> (-72.6154, -86.4272)
  line L498 (-72.6154, -86.4272) -> (-72.2665, -86.4274)
  line L499 (-72.2665, -86.4274) -> (-71.9175, -86.4277)
  line L500 (-71.9175, -86.4277) -> (-71.9137, -86.9611)
  line L501 (-71.9137, -86.9611) -> (-71.9031, -87.3722)
  line L502 (-71.9031, -87.3722) -> (-71.8747, -87.5388)
  line L503 (-71.8747, -87.5388) -> (-71.8521, -87.5327)
  line L504 (-71.8521, -87.5327) -> (-71.8229, -87.4679)
  line L505 (-71.8229, -87.4679) -> (-71.742, -87.1663)
  line L506 (-71.742, -87.1663) -> (-71.6615, -86.8618)
  line L507 (-71.6615, -86.8618) -> (-71.5825, -86.6242)
  line L508 (-71.5825, -86.6242) -> (-71.5192, -86.4907)
  line L509 (-71.5192, -86.4907) -> (-71.498, -86.4748)
  line L510 (-71.498, -86.4748) -> (-71.4861, -86.4988)
  line L511 (-71.4861, -86.4988) -> (-71.5081, -86.8047)
  line L512 (-71.5081, -86.8047) -> (-71.5939, -87.306)
  line L513 (-71.5939, -87.306) -> (-71.7083, -87.8237)
  line L514 (-71.7083, -87.8237) -> (-71.8163, -88.1789)
  line L515 (-71.8163, -88.1789) -> (-71.9579, -88.5788)
  line L516 (-71.9579, -88.5788) -> (-72.0241, -88.7534)
  line L517 (-72.0241, -88.7534) -> (-72.0484, -88.791)
  line L518 (-72.0484, -88.791) -> (-72.0634, -88.7882)
  line L519 (-72.0634, -88.7882) -> (-72.0634, -88.7883)
  line L520 (-69.0039, -88.4741) -> (-69.0042, -88.1028)
  line L521 (-69.0042, -88.1028) -> (-70.2811, -88.1028)
  line L522 (-70.2811, -88.1028) -> (-71.1064, -88.1018)
  line L523 (-71.1064, -88.1018) -> (-71.3446, -88.0918)
  line L524 (-71.3446, -88.0918) -> (-71.492, -88.0678)
  line L525 (-71.492, -88.0678) -> (-71.5676, -88.0238)
  line L526 (-71.5676, -88.0238) -> (-71.5906, -87.9542)
  line L527 (-71.5906, -87.9542) -> (-71.5551, -87.7145)
  line L528 (-71.5551, -87.7145) -> (-71.463, -86.9508)
  line L529 (-71.463, -86.9508) -> (-71.3968, -86.4459)
  line L530 (-71.3968, -86.4459) -> (-69.0318, -86.4364)
  line L531 (-69.0318, -86.4364) -> (-66.6863, -86.4462)
  line L532 (-66.6863, -86.4462) -> (-67.2057, -86.9984)
  line L533 (-67.2057, -86.9984) -> (-68.3644, -88.198)
  line L534 (-68.3644, -88.198) -> (-69.0036, -88.8454)
  line L535 (-69.0036, -88.8454) -> (-69.0039, -88.4741)
  line L536 (-4.5118, -87.7375) -> (-4.1854, -87.4352)
  line L537 (-4.1854, -87.4352) -> (-3.9561, -87.2705)
  line L538 (-3.9561, -87.2705) -> (-3.8548, -87.2276)
  line L539 (-3.8548, -87.2276) -> (-3.75, -87.2044)
  line L540 (-3.75, -87.2044) -> (-3.4935, -87.1977)
  line L541 (-3.4935, -87.1977) -> (-3.2907, -87.1934)
  line L542 (-3.2907, -87.1934) -> (-3.2304, -87.1765)
  line L543 (-3.2304, -87.1765) -> (-3.1947, -87.1453)
  line L544 (-3.1947, -87.1453) -> (-3.1814, -87.0961)
  line L545 (-3.1814, -87.0961) -> (-3.1885, -87.0257)
  line L546 (-3.1885, -87.0257) -> (-3.2553, -86.8072)
  line L547 (-3.2553, -86.8072) -> (-3.2881, -86.7054)
  line L548 (-3.2881, -86.7054) -> (-3.297, -86.6288)
  line L549 (-3.297, -86.6288) -> (-3.2699, -86.5741)
  line L550 (-3.2699, -86.5741) -> (-3.1949, -86.5382)
  line L551 (-3.1949, -86.5382) -> (-3.0599, -86.5178)
  line L552 (-3.0599, -86.5178) -> (-2.8529, -86.5098)
  line L553 (-2.8529, -86.5098) -> (-2.175, -86.5177)
  line L554 (-2.175, -86.5177) -> (-0.6138, -86.5397)
  line L555 (-0.6138, -86.5397) -> (-0.2562, -86.5429)
  line L556 (-0.2562, -86.5429) -> (-0.1577, -86.5575)
  line L557 (-0.1577, -86.5575) -> (-0.1056, -86.5913)
  line L558 (-0.1056, -86.5913) -> (-0.0948, -86.652)
  line L559 (-0.0948, -86.652) -> (-0.1201, -86.7476)
  line L560 (-0.1201, -86.7476) -> (-0.2581, -87.0745)
  line L561 (-0.2581, -87.0745) -> (-0.3916, -87.3459)
  line L562 (-0.3916, -87.3459) -> (-0.5564, -87.6321)
  line L563 (-0.5564, -87.6321) -> (-0.7067, -87.8584)
  line L564 (-0.7067, -87.8584) -> (-0.7965, -87.9504)
  line L565 (-0.7965, -87.9504) -> (-0.8249, -87.9106)
  line L566 (-0.8249, -87.9106) -> (-0.8498, -87.8046)
  line L567 (-0.8498, -87.8046) -> (-0.8759, -87.4744)
  line L568 (-0.8759, -87.4744) -> (-0.8939, -87.312)
  line L569 (-0.8939, -87.312) -> (-0.9347, -87.1888)
  line L570 (-0.9347, -87.1888) -> (-0.9653, -87.1516)
  line L571 (-0.9653, -87.1516) -> (-0.9809, -87.1907)
  line L572 (-0.9809, -87.1907) -> (-0.9799, -87.6172)
  line L573 (-0.9799, -87.6172) -> (-0.968, -88.1409)
  line L574 (-0.968, -88.1409) -> (-2.9493, -88.1406)
  line L575 (-2.9493, -88.1406) -> (-4.9307, -88.1403)
  line L576 (-4.9307, -88.1403) -> (-4.5118, -87.7375)
  line L577 (-45.3837, -84.2469) -> (-45.9444, -83.6852)
  line L578 (-45.9444, -83.6852) -> (-47.665, -83.6852)
  line L579 (-47.665, -83.6852) -> (-49.3855, -83.6852)
  line L580 (-49.3855, -83.6852) -> (-49.4444, -83.8471)
  line L581 (-49.4444, -83.8471) -> (-49.5486, -84.1803)
  line L582 (-49.5486, -84.1803) -> (-49.5755, -84.2743)
  line L583 (-49.5755, -84.2743) -> (-49.5853, -84.2926)
  line L584 (-49.5853, -84.2926) -> (-49.5942, -84.2893)
  line L585 (-49.5942, -84.2893) -> (-49.6427, -84.0242)
  line L586 (-49.6427, -84.0242) -> (-49.7702, -83.3811)
  line L587 (-49.7702, -83.3811) -> (-49.8432, -83.0646)
  line L588 (-49.8432, -83.0646) -> (-49.8384, -83.0396)
  line L589 (-49.8384, -83.0396) -> (-49.8098, -83.0759)
  line L590 (-49.8098, -83.0759) -> (-49.7947, -83.0729)
  line L591 (-49.7947, -83.0729) -> (-49.7877, -83.0056)
  line L592 (-49.7877, -83.0056) -> (-49.7975, -82.676)
  line L593 (-49.7975, -82.676) -> (-49.8265, -82.1132)
  line L594 (-49.8265, -82.1132) -> (-49.8204, -82.0518)
  line L595 (-49.8204, -82.0518) -> (-49.7803, -82.0063)
  line L596 (-49.7803, -82.0063) -> (-49.6803, -81.9594)
  line L597 (-49.6803, -81.9594) -> (-49.4947, -81.8942)
  line L598 (-49.4947, -81.8942) -> (-49.272, -81.8288)
  line L599 (-49.272, -81.8288) -> (-48.9695, -81.7952)
  line L600 (-48.9695, -81.7952) -> (-48.3819, -81.7829)
  line L601 (-48.3819, -81.7829) -> (-47.3038, -81.7811)
  line L602 (-47.3038, -81.7811) -> (-45.4479, -81.7811)
  line L603 (-45.4479, -81.7811) -> (-44.7445, -82.5153)
  line L604 (-44.7445, -82.5153) -> (-43.3367, -83.9846)
  line L605 (-43.3367, -83.9846) -> (-42.6199, -84.7535)
  line L606 (-42.6199, -84.7535) -> (-42.9305, -84.7807)
  line L607 (-42.9305, -84.7807) -> (-43.7152, -84.798)
  line L608 (-43.7152, -84.798) -> (-44.8229, -84.8087)
  line L609 (-44.8229, -84.8087) -> (-45.3837, -84.2469)
  line L610 (-49.2459, -82.1048) -> (-49.249, -81.8382)
  line L611 (-49.249, -81.8382) -> (-49.2981, -82.181)
  line L612 (-49.2981, -82.181) -> (-49.3487, -82.6669)
  line L613 (-49.3487, -82.6669) -> (-49.345, -82.705)
  line L614 (-49.345, -82.705) -> (-49.3348, -82.7049)
  line L615 (-49.3348, -82.7049) -> (-49.295, -82.5808)
  line L616 (-49.295, -82.5808) -> (-49.259, -82.3546)
  line L617 (-49.259, -82.3546) -> (-49.2459, -82.1048)
  point P0 (0, 0)
  point P1 (-3.7121, -94.6461)
  point P2 (-72.0634, -88.7882)
  constraints: 1236 end point
extrude "Extrusion2" cut sketch "Sketch2" against normal blind 3
sketch "Sketch5" plane through (0, 10, 0) normal (0, 1, 0) x (1, 0, 0)
  circle A0 centre (-102.5, -90) radius 3.3
  line L0 (-112.5, 100) -> (-112.5, -100) projected
  line L1 (-112.5, -100) -> (112.5, -100) projected
  circle A1 centre (-102.5, 72) radius 3.3
  line L2 (112.5, 100) -> (-112.5, 100) projected
  circle A2 centre (102.5, 90) radius 3.3
  circle A3 centre (102.5, -90) radius 3.3
  line L3 (112.5, -100) -> (112.5, 100) projected
  point P0 (0, 0)
  dimension "d21" = 6.6
  dimension "d22" = 10
  dimension "d23" = 10
  dimension "d24" = 10
  dimension "d25" = 28
  dimension "d26" = 10
  dimension "d27" = 10
  dimension "d28" = 10
  dimension "d29" = 10
  constraints: 4 centre point, 3 equal radius
  measures "d21" diameter of A0
  measures "d22" distance from line of L0 A0.centre
  measures "d23" distance from line of L1 A0.centre
  measures "d24" distance from line of L0 A1.centre
  measures "d25" distance from line of L2 A1.centre
  measures "d26" distance from line of L2 A2.centre
  measures "d27" distance from line of L3 A2.centre
  measures "d28" distance from line of L1 A3.centre
  measures "d29" distance from line of L3 A3.centre
extrude "Extrusion5" cut sketch "Sketch5" against normal blind 10 contours A0 | A1 | A2 | A3
body "Solid1"
